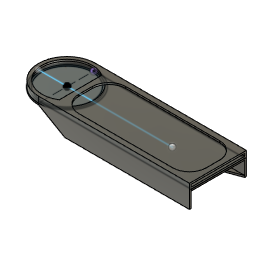
QuestSideLabelHolder (Autodesk Fusion 360 design; units mm, degrees)
Autodesk Fusion 360 part; units mm, degrees
note: some values were not read from the file. Chosen so that the rebuilt part matches the saved one: which bodies a step acts on; which face or edge a step refers to; the sign of a taper. Set by a fixed rule: which sketch regions a step uses.
sketch "Esquisse1" plane through (0, 0, 0) normal (0, 0, 1) x (1, 0, 0)
  line L0 (0, 0) -> (90, 0)
  line L1 (90, 0) -> (90, -32)
  line L2 (90, -32) -> (0, -32)
  line L3 (0, -32) -> (0, 0) construction
  circle A0 centre (0, -16) radius 16
  circle A1 centre (0, -16) radius 15
  circle A2 centre (0, -16) radius 17
  dimension "d1" = 90
  dimension "d2" = 32
  dimension "d12" = -1
  dimension "d13" = 1
  constraint horizontal L0
  constraint vertical L1
  constraint horizontal L2
  constraint vertical L3
  constraint coincident L0.start L3.end
  constraint midpoint L3 A0.centre
  constraint coincident L0.start A0
  measures "d1" distance of L0.start L0.end
  measures "d2" distance of L0.start L2.end
sketch "Esquisse2" plane through (0, 0, 0) normal (1, 0, 0) x (0, 1, 0)
  line L0 (0, 0) -> (-32, 0)
  line L1 (-32, 0) -> (-32, -9)
  line L2 (0, -9) -> (0, 0)
  circle A0 centre (-16, -9) radius 4 construction
  line L3 (-32, -9) -> (-20, -9)
  line L4 (-12, -9) -> (0, -9)
  line L5 (-12, -10) -> (1, -10)
  line L6 (1, -10) -> (1, 1)
  line L7 (1, 1) -> (-33, 1)
  line L8 (-33, 1) -> (-33, -10)
  line L9 (-33, -10) -> (-20, -10)
  line L10 (-20, -10) -> (-20, -9)
  line L11 (-12, -10) -> (-12, -9)
  line L12 (-33, 1) -> (1, 1)
  line L13 (1, 1) -> (1, 3.5)
  line L14 (1, 3.5) -> (-33, 3.5)
  line L15 (-33, 3.5) -> (-33, 1)
  line L16 (0, 2) -> (0, 2.5)
  line L17 (0, 2.5) -> (-32, 2.5)
  line L18 (-32, 2.5) -> (-32, 2)
  line L19 (-32, 2) -> (-32, 1)
  line L20 (0, 2) -> (0, 1)
  line L21 (-32, 2.5) -> (-32, 3.5)
  line L22 (0, 2.5) -> (0, 3.5)
  dimension "d3" = 9
  dimension "d4" = 8
  dimension "d5" = 1
  dimension "d6" = 2.5
  constraint horizontal L0
  constraint vertical L1
  constraint horizontal L3
  constraint vertical L2
  constraint coincident L0.start L2.end
  constraint coincident A0 L3.end
  constraint coincident A0 L4.start
  constraint collinear L3 L4
  constraint coincident A0.centre L3
  constraint tangent A0 L10
  constraint tangent A0 L11
  constraint horizontal L12
  constraint vertical L13
  constraint horizontal L14
  constraint vertical L15
  constraint coincident L12 L19.end
  constraint perpendicular L12 L19
  constraint coincident L7 L20.end
  constraint perpendicular L7 L20
  constraint coincident L14 L21.end
  constraint perpendicular L14 L21
  constraint coincident L14 L22.end
  constraint perpendicular L14 L22
  measures "d3" distance of L0.start L2.start
  measures "d4" diameter of A0
  measures "d6" distance of L7.end L14.end
extrude "Extrusion1" add sketch "Esquisse1" against normal blind 1 contours L0 L2 A0 A2 | A0 | L0 L1 L2 A2 | A1 picked at (5.633, -31.302) makes body 1
extrude "Extrusion2" add sketch "Esquisse2" along normal blind 90 contours L0 L1 L2 L3 L4 L5 L6 L7 L8 L9 L10 L11 L12 | L7 L12 L13 L14 L16 L20 L22 | L7 L12 L14 L15 L18 L19 L21 | L14 L17 L21 L22 bodies 1
extrude "Extrusion3" add sketch "Esquisse1" along normal blind 3.5 contours L0 L2 A0 A2 picked at (-16.3035, -16) bodies 1
extrude "Extrusion4" cut sketch "Esquisse1" along normal blind 5 contours A0 | A1 bodies 1
extrude "Extrusion5" add sketch "Esquisse1" against normal blind 1 contours L0 L2 A0 A2 | L0 L2 A0 A2 bodies 1
extrude "Extrusion6" add sketch "Esquisse1" along normal blind 1 separate body contours L0 L2 A0 A2 | A0 picked at (5.633, -31.302) makes body 2
move_body "Déplacer1" bodies 2 to x (1, 0, 0) y (0, 1, 0) z (0, 0, 1) at (0, 0, 2.5)
extrude "Extrusion7" add sketch "Esquisse2" along normal blind 80 separate body contours L14 L17 L21 L22 makes body 3
move_body "Déplacer2" bodies 3 to x (1, 0, 0) y (0, 1, 0) z (0, 0, 1) at (8, 0, 0)
draft "Dépouille1" angle 60 neutral plane through (0, 0, -1) pull (0, 0, -1) 1 faces at (0, -28.3333, -9.6667) on bodies 1
draft "Dépouille2" angle -60 neutral plane through (0, 0, -1) pull (0, 0, 1) 1 faces at (0, -3.6667, -9.6667) on bodies 1
sketch "Esquisse3" plane through (0, 0, 0) normal (0, 0, 1) x (1, 0, 0)
  line L0 (-17.3429, -15.9329) -> (62.6571, -15.9329)
  dimension "d31" = 80
  constraint horizontal L0
  measures "d31" distance of L0.start L0.end
extrude "Extrusion8" add sketch "Esquisse2" along normal blind 1 separate body contours L0 L1 L2 L3 L4 L5 L6 L7 L8 L9 L10 L11 L12 makes body 4
move_body "Déplacer3" bodies 4 to x (1, 0, 0) y (0, 1, 0) z (0, 0, 1) at (96, 0, 0)
extrude "Extrusion9" add 1 faces at (96.3333, -10.6667, 0) along direction (0, 0, -1) blind 1 on bodies 4 bodies 4
extrude "Extrusion10" cut 1 faces at (96.3333, -10.6667, -1) along direction (0, 0, 1) blind 4.5 on bodies 4 bodies 4 makes body 5 at (96, -28.3333, -9.6667)
sketch "Esquisse4" plane through (90, 0, 0) normal (1, 0, 0) x (0, 1, 0)
  line L0 (-32, 2.5) -> (0, 2.5)
  line L1 (0, 2.5) -> (0, 1)
  line L2 (0, 1) -> (-32, 1)
  line L3 (-32, 1) -> (-32, 2.5)
  line L4 (0, -1) -> (0, -9)
  line L5 (0, -9) -> (-12, -9)
  line L6 (-12, -9) -> (-12, -10)
  line L7 (-12, -10) -> (1, -10)
  line L8 (1, -10) -> (1, 3.5)
  line L9 (1, 3.5) -> (-33, 3.5)
  line L10 (-33, 3.5) -> (-33, -10)
  line L11 (-33, -10) -> (-20, -10)
  line L12 (-20, -10) -> (-20, -9)
  line L13 (-20, -9) -> (-32, -9)
  line L14 (-32, -9) -> (-32, -1)
  line L15 (-32, -1) -> (0, -1)
  line L16 (0, -9) -> (-12, -9)
  line L17 (-12, -9) -> (-12, -10)
  line L18 (-12, -10) -> (0, -10)
  line L19 (0, -10) -> (0, -9)
  line L20 (-20, -9) -> (-32, -9)
  line L21 (-32, -9) -> (-32, -10)
  line L22 (-32, -10) -> (-20, -10)
  line L23 (-20, -10) -> (-20, -9)
  constraint horizontal L16
  constraint vertical L17
  constraint horizontal L18
  constraint vertical L19
  constraint coincident L6.end L7.start
  constraint coincident L4.end L5.start
  constraint horizontal L20
  constraint vertical L21
  constraint horizontal L22
  constraint vertical L23
  constraint coincident L11 L21.end
  constraint coincident L12.end L13.start
extrude "Extrusion11" cut sketch "Esquisse4" against normal blind 0.01 contours L5 L6 L7 L16 L17 L18 L19 | L11 L12 L13 L20 L21 L22 L23 bodies 1
draft "Dépouille3" angle 70 neutral plane through (0, -32, 0) pull (0, 1, 0) 1 faces at (89.99, -28, -9.6667) on bodies 1
draft "Dépouille4" angle 70 neutral plane through (0, 0, -9) pull (0, -1, 0) 1 faces at (89.99, -4, -9.6667) on bodies 1
sketch "Esquisse5" plane through (0, 0, 3.5) normal (0, 0, 1) x (-1, 0, 0)
  circle A0 centre (0, 16) radius 16
  line L0 (0, 33) -> (-90, 33)
  line L1 (-90, 33) -> (-90, -1)
  line L2 (-90, -1) -> (0, -1)
  arc A1 (0, -1) -> (0, 33) centre (0, 16) ccw
  line L3 (-90, 33) -> (-8, 33)
  line L4 (-8, 33) -> (-8, -1)
  line L5 (-8, -1) -> (-90, -1)
  line L6 (-90, -1) -> (-90, 33)
  line L7 (-87, 12) -> (-87, 20)
  line L8 (-77, 30) -> (-21, 30)
  line L9 (-11, 20) -> (-11, 12)
  line L10 (-21, 2) -> (-77, 2)
  arc A2 (-21, 2) -> (-11, 12) centre (-21, 12) ccw
  arc A3 (-11, 20) -> (-21, 30) centre (-21, 20) ccw
  arc A4 (-87, 12) -> (-77, 2) centre (-77, 12) ccw
  arc A5 (-77, 30) -> (-87, 20) centre (-77, 20) ccw
  dimension "d45" = 10
  constraint horizontal L3
  constraint vertical L4
  constraint horizontal L5
  constraint vertical L6
  constraint coincident L2 L4.end
  constraint coincident L0.end L1.start
  constraint tangent L9 A2
  constraint tangent L10 A2
  constraint tangent L9 A3
  constraint tangent L8 A3
  constraint equal A2 A3
  constraint tangent L10 A4
  constraint tangent L7 A4
  constraint equal A2 A4
  constraint tangent L7 A5
  constraint tangent L8 A5
  constraint equal A2 A5
  measures "d45" radius of A2
extrude "Extrusion12" cut sketch "Esquisse5" against normal blind 1.1 contours A0 L9 A2 A3 | A0 L7 L8 L10 A2 A3 A4 A5 bodies 1 2 3
combine "Combiner1" operation add target body 1 tool bodies 3
combine "Combiner2" operation add target body 2 tool bodies 1
hidden bodies 4 5
